Autodesk Fusion 360 part; units mm, degrees
(part 3 of 3)
  line L1766 (-132.0556, -11.6036) -> (-130.7565, -10.8536)
  line L1767 (-169.1667, -11.6036) -> (-167.8676, -10.8536)
  line L1768 (-143.1667, -11.6036) -> (-141.8676, -10.8536)
  line L1769 (-155.0158, -19.1686) -> (-156.3148, -18.4186)
  line L1770 (-162.4232, -20.6686) -> (-162.4232, -19.1686)
  line L1771 (-139.8121, 0.75) -> (-141.1111, 1.5)
  line L1772 (-152.2222, 1.5) -> (-153.5213, 0.75)
  line L1773 (-136.0343, 0.75) -> (-137.3333, 1.5)
  line L1774 (-147.2195, 0.75) -> (-148.5185, 1.5)
  line L1775 (-129.9259, 1.5) -> (-131.225, 0.75)
  line L1776 (-163.0583, -10.8536) -> (-161.7593, -11.6036)
  line L1777 (-120.9444, -11.6036) -> (-119.6454, -10.8536)
  line L1778 (-189.0583, -10.8536) -> (-187.7593, -11.6036)
  line L1779 (-184.3306, 0.75) -> (-185.6296, 1.5)
  line L1780 (-181.9259, 1.5) -> (-183.225, 0.75)
  line L1781 (-128.3519, -11.6036) -> (-127.0528, -10.8536)
  line L1782 (-135.7593, -11.6036) -> (-134.4602, -10.8536)
  line L1783 (-121.2195, 0.75) -> (-122.5185, 1.5)
  line L1784 (-180.6269, 0.75) -> (-181.9259, 1.5)
  line L1785 (-133.3546, -10.8536) -> (-132.0556, -11.6036)
  line L1786 (-154.3519, -11.6036) -> (-153.0528, -10.8536)
  line L1787 (-156.3148, -18.4186) -> (-157.6139, -19.1686)
  line L1788 (-184.0556, -11.6036) -> (-182.7565, -10.8536)
  line L1789 (-166.762, -10.8536) -> (-165.463, -11.6036)
  line L1790 (-181.6509, -10.8536) -> (-180.3519, -11.6036)
  line L1791 (-137.0583, -10.8536) -> (-135.7593, -11.6036)
  line L1792 (-167.1667, -8.1395) -> (-165.8676, -7.3895)
  line L1793 (-143.5158, 0.75) -> (-144.8148, 1.5)
  line L1794 (-174.2435, -10.8536) -> (-172.9444, -11.6036)
  line L1795 (-155.9259, 1.5) -> (-157.225, 0.75)
  line L1796 (-180.3519, -11.6036) -> (-179.0528, -10.8536)
  line L1797 (-158.0556, -11.6036) -> (-156.7565, -10.8536)
  line L1798 (-167.1111, 1.5) -> (-168.4101, 0.75)
  line L1799 (-124.6481, -11.6036) -> (-123.3491, -10.8536)
  line L1800 (-139.463, -11.6036) -> (-138.1639, -10.8536)
  line L1801 (-159.3546, -10.8536) -> (-158.0556, -11.6036)
  line L1802 (-174.299, -17.4932) -> (-173, -18.2432)
  line L1803 (-173, -15.2432) -> (-174.299, -15.9932)
  line L1804 (-161.3176, -20.6686) -> (-160.0185, -21.4186)
  line L1805 (-165.8676, -5.8895) -> (-167.1667, -5.1395)
  line L1806 (-177.0528, -5.8895) -> (-178.3519, -5.1395)
  line L1807 (-165.5926, -15.2432) -> (-166.8916, -15.9932)
  line L1808 (-189.3333, 0) -> (-189.3333, -1.5)
  line L1809 (-189.3333, 0) -> (-29.3333, 0)
  line L1810 (-29.3333, 0) -> (-29.3333, -22)
  line L1811 (-29.3333, -22) -> (-189.3333, -22)
  line L1812 (-189.3333, -22) -> (-189.3333, 0)
  point P0 (-78, 0)
  point P1 (-78, 1.75)
  point P2 (-156, 0)
  point P3 (-156, 1.75)
  dimension "d34" = 160
  dimension "d35" = 22
  constraint vertical L1808
  constraint horizontal L1809
  constraint vertical L1812
  constraint coincident L1809 L1687.end
  measures "d34" distance of L1808.start L1809.end
  measures "d35" distance of L1808.start L1811.end
sketch "Sketch2" plane through (0, 0, 0) normal (0, 0, 1) x (1, 0, 0)
extrude "Extrude1" add sketch "Sketch1" along normal blind 3 contours L3 L4 L5 L8 L203 L219 L223 L226 L230 L236 L249 L250 L258 L266 L277 L280 L302 L303 L330 L411 L424 L461 L509 L537 L538 L593 L595 L597 L600 L609 L635 L639 L643 L648 L680 L699 L704 L706 L713 L721 L723 L742 L752 L763 L769 L787 L792 L793 L796 L798 L802 L803 L804 L805 L814 L824 L830 L832 L839 L841 L844 L845 L848 L849 L856 L861 L862 L864 L868 L876 L887 L893 L895 L896 L898 L899 L900 L905 L910 L922 L924 L925 L926 L928 L933 L935 L938 L957 L1021 L1058 L1079 L1084 L1099 L1103 L1106 L1110 L1116 L1129 L1130 L1138 L1146 L1157 L1160 L1168 L1182 L1183 L1210 L1291 L1304 L1341 L1389 L1417 L1418 L1473 L1475 L1477 L1480 L1489 L1506 L1514 L1518 L1522 L1527 L1559 L1578 L1583 L1585 L1592 L1600 L1602 L1621 L1631 L1642 L1648 L1658 L1660 L1664 L1666 L1667 L1668 L1669 L1670 L1671 L1672 L1673 L1675 L1677 L1679 L1680 L1683 L1684 L1685 L1686 L1687 L1688 L1689 L1691 L1692 L1694 L1695 L1696 L1699 L1700 L1701 L1702 L1704 L1705 L1706 L1710 L1714 L1726 L1728 L1729 L1730 L1732 L1733 L1734 L1735 L1754 L1809 L1810 L1811 L1812
